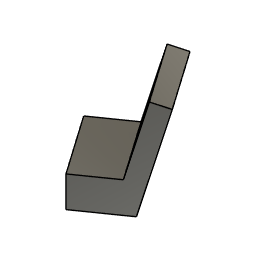
cam_holder v2 (Autodesk Fusion 360 design; units mm, degrees)
Autodesk Fusion 360 part; units mm, degrees
sketch "Sketch4" plane through (0, 0, 0) normal (0, 0, -1) x (1, 0, 0)
  line L0 (14.5, -60) -> (8, -60)
  line L1 (8, -60) -> (8, -48)
  line L2 (8, -48) -> (14.5, -48)
  line L3 (0, -80) -> (18.5, -80)
  line L4 (102.7523, -51.9047) -> (127.501, -76.6535)
  line L5 (-102.7523, -51.9047) -> (-122.8275, -80.5751)
  line L6 (102.7523, -51.9047) -> (127.501, -76.6535)
  line L7 (127.501, -76.6535) -> (133.1579, -70.9966)
  line L8 (133.1579, -70.9966) -> (108.4092, -46.2479)
  line L9 (108.4092, -46.2479) -> (102.7523, -51.9047)
  line L10 (-122.8275, -80.5751) -> (-102.7523, -51.9047)
  line L11 (-102.7523, -51.9047) -> (-109.3055, -47.3161)
  line L12 (-109.3055, -47.3161) -> (-129.3807, -75.9864)
  line L13 (-129.3807, -75.9864) -> (-122.8275, -80.5751)
  circle A0 centre (11, -76) radius 1.5
  circle A1 centre (11, -36) radius 1.5
  dimension "d122" = 35
  dimension "d124" = 35
  dimension "d125" = 8
  dimension "d126" = 8
  constraint perpendicular L6 L7
  constraint parallel L6 L8
  constraint parallel L7 L9
  constraint perpendicular L10 L11
  constraint parallel L10 L12
  constraint parallel L11 L13
  measures "d122" distance of L4.start L4.end
  measures "d124" distance of L5.start L5.end
  measures "d125" distance of L4.start L8.end
  measures "d126" distance of L5.end L12.end
extrude "Extrude15" add sketch "Sketch4" against normal blind 15 contours L5 L10 L11 L12 L13 in component "Base"
sketch "Sketch6" plane through (-78.2669, 111.7767, 0) normal (-0.573576, 0.819152, 0) x (-0.819152, -0.573576, 0)
  line L0 (54.3984, 0) -> (62.3984, 0)
  line L1 (62.3984, 0) -> (62.3984, 15)
  line L2 (62.3984, 15) -> (54.3984, 15)
  line L3 (54.3984, 15) -> (54.3984, 0)
  line L4 (62.3984, 15) -> (54.3984, 12.8564)
  line L5 (62.3984, 15) -> (70.6806, 15) construction
  dimension "d131" = 165
  constraint horizontal L5
  constraint coincident L1.end L2.start
  constraint coincident L3 L4.end
  measures "d131" angle of L4 L5
extrude "Extrude17" cut sketch "Sketch6" against normal up to surface (35 mm away) contours L2 L3 L4 in component "Base"
extrude "Extrude19" add 1 faces at (-113.8128, 58.4024, 14.2855) along direction (0.212012, 0.148453, 0.965926) blind 35 in component "Base"
sketch "Sketch8" plane through (-50.7617, -35.5437, 16.6044) normal (-0.79124, -0.554032, 0.258819) x (0.573576, -0.819152, 0)
  line L0 (-136.4542, -1.661) -> (-101.4542, -1.661)
  line L1 (-101.4542, -1.661) -> (-101.4542, 33.339)
  line L2 (-101.4542, 33.339) -> (-136.4542, 33.339)
  line L3 (-136.4542, 33.339) -> (-136.4542, -1.661)
  line L4 (-136.4542, 15.839) -> (-101.4542, 15.839)
  line L5 (-111.4542, 8.339) -> (-126.4542, 8.339)
  line L6 (-126.4542, 8.339) -> (-126.4542, 23.339)
  line L7 (-126.4542, 23.339) -> (-111.4542, 23.339)
  line L8 (-111.4542, 23.339) -> (-111.4542, 8.339)
  line L9 (-111.4542, 8.339) -> (-126.4542, 23.339) construction
  line L10 (-126.4542, 8.339) -> (-111.4542, 23.339) construction
  line L11 (-105.4542, 12.839) -> (-132.4542, 12.839)
  line L12 (-132.4542, 12.839) -> (-132.4542, 18.839)
  line L13 (-132.4542, 18.839) -> (-105.4542, 18.839)
  line L14 (-105.4542, 18.839) -> (-105.4542, 12.839)
  line L15 (-105.4542, 12.839) -> (-132.4542, 18.839) construction
  line L16 (-132.4542, 12.839) -> (-105.4542, 18.839) construction
  circle A0 centre (-118.9542, 15.839) radius 7.5
  circle A1 centre (-134.9542, 31.839) radius 1
  circle A2 centre (-134.9542, -0.161) radius 1
  circle A3 centre (-102.9542, -0.161) radius 1
  circle A4 centre (-102.9542, 31.839) radius 1
  point P0 (-118.9542, 15.839)
  point P1 (-118.9542, 15.839)
  dimension "d141" = 15
  dimension "d142" = 15
  dimension "d143" = 27
  dimension "d144" = 6
  dimension "d149" = 2
  dimension "d150" = 1.5
  dimension "d151" = 1.5
  dimension "d153" = 360
  constraint midpoint L3 L4.start
  constraint midpoint L1 L4.end
  constraint horizontal L5
  constraint perpendicular L5 L6
  constraint parallel L5 L7
  constraint parallel L6 L8
  constraint coincident L9 P1
  constraint coincident L10 P1
  constraint midpoint L4 P1
  constraint horizontal L11
  constraint perpendicular L11 L12
  constraint parallel L11 L13
  constraint parallel L12 L14
  constraint coincident L15 P1
  constraint coincident L16 P1
  constraint coincident P1 P0
  constraint tangent L8 A0
  measures "d141" distance of L6.end L7.end
  measures "d142" distance of L5.end L6.end
  measures "d143" distance of L12.end L13.end
  measures "d144" distance of L11.end L12.end
  measures "d149" diameter of A1
  measures "d150" distance of L2 A1.centre
  measures "d151" distance of L3 A1.centre
extrude "Extrude20" cut sketch "Sketch8" against normal blind 5 contours L4 L6 L12 L13 | L4 L6 L11 L12 | L4 L8 L11 L14 | L4 L8 L13 L14 | L4 L13 A0 | L6 L11 A0 | L6 L13 A0 | L4 L11 A0 | L8 L13 A0 | L8 L11 A0 | L5 L6 L11 A0 | L6 L7 L13 A0 | L13 A0 | L11 A0 | L7 L8 L13 A0 | L5 L8 L11 A0 in component "Base"
extrude "Extrude21" cut sketch "Sketch8" against normal up to surface (8.2822 mm away) contours L4 L13 A0 | L4 L11 A0 | L13 A0 | L11 A0 in component "Base"
extrude "Extrude22" cut sketch "Sketch8" against normal blind 4 contours A1 | A2 | A3 | A4 in component "Base"
extrude "Extrude23" add 1 faces at (-122.689, 66.4297, 10) along direction (-0.819152, -0.573576, 0) blind 20 in component "Base"
sketch "Sketch10" plane through (-78.2669, 111.7767, 0) normal (-0.573576, 0.819152, 0) x (-0.819152, -0.573576, 0)
  line L0 (54.3984, 12.8564) -> (54.3984, 0)
  line L1 (54.3984, 0) -> (82.3984, 0)
  line L2 (82.3984, 0) -> (82.3984, 15)
  line L3 (82.3984, 15) -> (62.3984, 15)
  line L4 (62.3984, 15) -> (53.3398, 48.8074)
  line L5 (53.3398, 48.8074) -> (45.3398, 46.6638)
  line L6 (45.3398, 46.6638) -> (54.3984, 12.8564)
  line L7 (45.3398, 46.6638) -> (57.8433, 0)
  constraint coincident L5.end L6.start
  constraint coincident L1 L7.end
  constraint perpendicular L5 L7
extrude "Extrude25" cut sketch "Sketch10" against normal up to surface (35 mm away) contours L0 L1 L7 in component "Base"
component "Base" placed x (1, 0, 0) y (0, 1, 0) z (0, 0, 1) at (0, 0, 0)
named bodies: "cam-side-mnt1"
